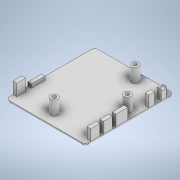
# Autodesk Inventor part: Part1
Saved by Autodesk Inventor 2022 (Build 260153000, 153)
## iProperties
Created: 2021-10-11
Part Number: Part1
Material: Generic
Document SubType Name: Modeling
Designer: Route
Density: 1 g/cm^3
Appearance: Default
Author: Route
Autodesk Inventor part; units mm, degrees
ref_plane "YZ Plane" through (0, 0, 0) normal (1, 0, 0) x (0, 1, 0)
ref_plane "XZ Plane" through (0, 0, 0) normal (0, 1, 0) x (-1, 0, 0)
ref_plane "XY Plane" through (0, 0, 0) normal (0, 0, 1) x (1, 0, 0)
sketch "Sketch1" plane through (0, 0, 0) normal (0, 1, 0) x (-1, 0, 0)
  line L0 (-30, -34) -> (30, -34)
  line L1 (30, -34) -> (30, 34)
  line L2 (30, 34) -> (-30, 34)
  line L3 (-30, 34) -> (-30, -34)
  line L4 (-30, -34) -> (30, 34) construction
  line L5 (30, -34) -> (-30, 34) construction
  line L6 (-33, 37) -> (33, 37)
  line L7 (33, 37) -> (33, -37)
  line L8 (33, -37) -> (-33, -37)
  line L9 (-33, -37) -> (-33, 37)
  line L10 (-33, 37) -> (33, -37) construction
  line L11 (33, 37) -> (-33, -37) construction
  point P0 (0, 0)
  dimension "d0" = 66
  dimension "d1" = 74
  constraints: 24 end point, 4 midpoint, 4 parallel, 2 horizontal, 2 perpendicular
  measures "d0" distance of L7.end L8.end
  measures "d1" distance of L6.end L7.end
extrude "Extrusion1" add sketch "Sketch1" along normal blind 3 contours L3 L2 L1 L0 | L6 L7 L8 L9
sketch "Sketch2" plane through (0, 3, 0) normal (0, 1, 0) x (1, 0, 0)
  line L0 (30, -34) -> (-30, -34)
  line L1 (-30, -34) -> (-30, 34)
  line L2 (-30, 34) -> (30, 34)
  line L3 (30, 34) -> (30, -34)
  line L4 (30, -34) -> (-30, 34) construction
  line L5 (-30, -34) -> (30, 34) construction
  line L6 (33, 37) -> (-33, 37) projected
  line L7 (33, -37) -> (-33, -37)
  line L8 (-33, -37) -> (-33, 37)
  line L9 (-33, 37) -> (33, 37)
  line L10 (33, 37) -> (33, -37)
  line L11 (33, -37) -> (-33, 37) construction
  line L12 (-33, -37) -> (33, 37) construction
  point P0 (0, 0)
  constraints: 24 end point, 4 midpoint, 4 parallel, 2 horizontal, 2 perpendicular
extrude "Extrusion2" add sketch "Sketch2" along normal blind 15
fillet "Fillet1" radius 3 4 edges at (33, 9, 37) (33, 9, -37) (-33, 9, -37) (-33, 9, 37)
fillet "Fillet2" radius 3 8 edges at (-32.1213, 0, 36.1213) (0, 0, 37) (32.1213, 0, 36.1213) (33, 0, 0) (32.1213, 0, -36.1213) (0, 0, -37) (-32.1213, 0, -36.1213) (-33, 0, 0)
sketch "Sketch3" plane through (0, 3, 0) normal (0, 1, 0) x (1, 0, 0)
  arc A0 (33, 34) -> (30, 37) centre (30, 34) ccw projected
  circle A1 centre (8.41, 30.19) radius 1.5
  line L0 (30, 37) -> (30, 34) projected
  circle A2 centre (26.19, 6.06) radius 1.5
  line L1 (-30, -34) -> (30, -34) projected
  circle A3 centre (-3.25, -27.65) radius 1.5
  circle A4 centre (8.41, 30.19) radius 3
  circle A5 centre (-3.25, -27.65) radius 3
  circle A6 centre (26.19, 6.06) radius 3
  point P0 (0, 0)
  dimension "d10" = 3
  dimension "d13" = 3
  dimension "d16" = 3
  dimension "d17" = 6
  dimension "d18" = 6
  dimension "d19" = 6
  constraints: 6 centre point, 3 coincident
  measures "d10" diameter of A1
  measures "d13" diameter of A2
  measures "d16" diameter of A3
  measures "d17" diameter of A4
  measures "d18" diameter of A5
  measures "d19" diameter of A6
extrude "Extrusion3" add sketch "Sketch3" along normal blind 11.4
sketch "Sketch4" plane through (0, 3, 0) normal (0, 1, 0) x (1, 0, 0)
  circle A0 centre (8.41, 30.19) radius 1.5 projected
  circle A1 centre (8.41, 30.19) radius 1.5
  circle A2 centre (26.19, 6.06) radius 1.5 projected
  circle A3 centre (26.19, 6.06) radius 1.5
  circle A4 centre (-3.25, -27.65) radius 1.5 projected
  circle A5 centre (-3.25, -27.65) radius 1.5
  point P0 (0, 0)
  constraints: 3 centre point, 3 coincident
extrude "Extrusion4" cut sketch "Sketch4" against normal blind 3
sketch "Sketch5" plane through (0, 0, 0) normal (0, -1, 0) x (1, 0, 0)
  circle A0 centre (8.41, -30.19) radius 1.5 projected
  circle A1 centre (8.41, -30.19) radius 3
  circle A2 centre (26.19, -6.06) radius 1.5 projected
  circle A3 centre (26.19, -6.06) radius 3
  circle A4 centre (-3.25, 27.65) radius 3 projected
  circle A5 centre (-3.25, 27.65) radius 3
  point P0 (0, 0)
  dimension "d24" = 6
  constraints: 3 centre point, 3 coincident
  measures "d24" diameter of A1
extrude "Extrusion5" cut sketch "Sketch5" against normal blind 2
sketch "Sketch6" plane through (-30, 3, 34) normal (1, 0, 0) x (0, 0, -1)
  line L0 (0, 0) -> (68, 0) projected
  line L1 (0, 0) -> (0, 3.6)
  line L2 (0, 15) -> (0, 0) projected
  line L3 (0, 15) -> (68, 15) projected
  line L4 (68, 0) -> (0, 0) projected
  line L5 (14.69, 3) -> (25.84, 3)
  line L6 (14.69, 3) -> (14.69, 0)
  line L7 (25.84, 3) -> (25.84, 0)
  line L8 (9.91, 0) -> (9.91, 9.529)
  line L9 (2.79, 0) -> (2.79, 9.529)
  line L10 (2.79, 9.529) -> (9.91, 9.529)
  line L11 (10.16, 0) -> (14.44, 0)
  line L12 (26.09, 0) -> (68, 0)
  line L13 (68, 0) -> (68, 15) projected
  line L14 (68, 0) -> (68, 15)
  line L15 (-3, 15) -> (0, 15) projected
  line L16 (68, 15) -> (0, 15)
  line L17 (2.54, 0) -> (2.79, 0)
  line L18 (2.54, 0) -> (2.79, 0) construction
  line L19 (10.16, 0) -> (9.91, 0)
  line L20 (10.16, 0) -> (10.41, 0) construction
  line L21 (14.44, 0) -> (14.69, 0)
  line L22 (14.44, 0) -> (14.69, 0) construction
  line L23 (26.09, 0) -> (25.84, 0)
  line L24 (26.09, 0) -> (26.34, 0) construction
  point P0 (34, -3)
  point P1 (2.79, 0)
  dimension "d27" = 3.6
  dimension "d101" = 0.25
  dimension "d102" = 0
  dimension "d103" = 0.25
  dimension "d104" = 180
  dimension "d105" = 0.25
  dimension "d106" = 0
  dimension "d107" = 0.25
  dimension "d108" = 180
  constraints: 38 end point, 8 collinear, 6 perpendicular, 4 horizontal, 2 vertical, 1 point on line
  measures "d27" distance of L0.start L1.end
  measures "d101" distance of L17.start L17.end
  measures "d102" distance between parallel lines of L17 L18
  measures "d103" distance of L19.start L19.end
  measures "d104" angle of L19 L20
  measures "d105" distance of L21.start L21.end
  measures "d106" distance between parallel lines of L21 L22
  measures "d107" distance of L23.start L23.end
  measures "d108" angle of L23 L24
sketch "Sketch7" plane through (30, 3, -34) normal (-1, 0, 0) x (0, 0, 1)
  line L0 (68, 0) -> (0, 0) projected
  line L1 (68, 0) -> (68, 3.6)
  line L2 (68, 0) -> (68, 15) projected
  line L3 (66.48, 8.861) -> (59.24, 8.861)
  line L4 (49.08, 8.861) -> (56.32, 8.861)
  line L5 (36.5, 8.861) -> (46.16, 8.861)
  line L6 (0, 15) -> (0, 0) projected
  line L7 (0, 0) -> (0, 15) projected
  line L8 (0, 3.6) -> (2.29, 3.6) construction
  line L9 (0, 15) -> (68, 15) projected
  line L10 (36.25, 15) -> (46.41, 15)
  line L11 (48.83, 15) -> (56.57, 15)
  line L12 (59, 15) -> (66.73, 15)
  line L13 (9.39, 8.1692) -> (9.39, -1.0308)
  line L14 (5.39, 8.1692) -> (5.39, 0)
  line L15 (36.5, 8.861) -> (36.5, 0)
  line L16 (46.16, 8.861) -> (46.16, 0)
  line L17 (49.08, 8.861) -> (49.08, 0)
  line L18 (56.32, 8.861) -> (56.32, 0)
  line L19 (59.24, 8.861) -> (59.24, 0)
  line L20 (66.48, 8.861) -> (66.48, 0)
  line L21 (0, 0) -> (68, 0) projected
  line L22 (9.89, 0) -> (14.761, 0)
  line L23 (14.761, 0) -> (14.761, 8.861)
  line L24 (14.761, 8.861) -> (19.341, 8.861)
  line L25 (19.341, 8.861) -> (19.341, 0)
  line L26 (5.39, 0) -> (5.64, 0)
  line L27 (5.39, 0) -> (5.64, 0) construction
  line L28 (9.89, 0) -> (9.64, 0)
  line L29 (9.89, 0) -> (10.14, 0) construction
  line L30 (14.761, 0) -> (15.011, 0)
  line L31 (14.761, 0) -> (15.011, 0) construction
  line L32 (19.841, 0) -> (19.591, 0)
  line L33 (19.841, 0) -> (20.091, 0) construction
  arc A0 (5.39, 8.1692) -> (9.39, 8.1692) centre (7.39, 8.1692) ccw
  line L34 (36.25, 0) -> (36.5, 0)
  line L35 (36.25, 0) -> (36.5, 0) construction
  line L36 (46.41, 0) -> (46.16, 0)
  line L37 (46.41, 0) -> (46.66, 0) construction
  line L38 (48.83, 0) -> (49.08, 0)
  line L39 (48.83, 0) -> (49.08, 0) construction
  line L40 (56.57, 0) -> (56.32, 0)
  line L41 (56.57, 0) -> (56.82, 0) construction
  line L42 (58.99, 0) -> (59.24, 0)
  line L43 (58.99, 0) -> (59.24, 0) construction
  line L44 (66.73, 0) -> (66.48, 0)
  line L45 (66.73, 0) -> (66.98, 0) construction
  point P0 (34, -3)
  point P1 (66.48, 0)
  point P2 (5.39, 0)
  point P3 (9.39, 0)
  point P4 (19.341, 0)
  point P5 (9.39, 0)
  point P6 (66.48, 0)
  point P7 (19.341, 0)
  dimension "d70" = 9.2
  dimension "d78" = 4.871
  dimension "d80" = 90
  dimension "d81" = 0.25
  dimension "d82" = 0
  dimension "d83" = 0.25
  dimension "d84" = 180
  dimension "d85" = 0.25
  dimension "d86" = 0
  dimension "d87" = 0.25
  dimension "d88" = 180
  dimension "d89" = 0.25
  dimension "d90" = 0
  dimension "d91" = 0.25
  dimension "d92" = 180
  dimension "d93" = 0.25
  dimension "d94" = 0
  dimension "d95" = 0.25
  dimension "d96" = 180
  dimension "d97" = 0.25
  dimension "d98" = 0
  dimension "d99" = 0.25
  dimension "d100" = 180
  constraints: 80 end point, 17 collinear, 17 horizontal, 9 perpendicular, 3 point on line, 2 point on circle, 1 centre point, 1 parallel, 1 vertical, 1 other
  measures "d70" distance of L13.start L13.end
  measures "d78" distance of L22.start L22.end
  measures "d80" angle of L23 L24
  measures "d81" distance of L26.start L26.end
  measures "d82" distance between parallel lines of L26 L27
  measures "d83" distance of L28.start L28.end
  measures "d84" angle of L28 L29
  measures "d85" distance of L30.start L30.end
  measures "d86" distance between parallel lines of L30 L31
  measures "d87" distance of L32.start L32.end
  measures "d88" angle of L32 L33
  measures "d89" distance of L34.start L34.end
  measures "d90" distance between parallel lines of L34 L35
  measures "d91" distance of L36.start L36.end
  measures "d92" angle of L36 L37
  measures "d93" distance of L38.start L38.end
  measures "d94" distance between parallel lines of L38 L39
  measures "d95" distance of L40.start L40.end
  measures "d96" angle of L40 L41
  measures "d97" distance of L42.start L42.end
  measures "d98" distance between parallel lines of L42 L43
  measures "d99" distance of L44.start L44.end
  measures "d100" angle of L44 L45
ref_plane "Work Plane1" through (30, 3, -1) normal (0, 0, -1) x (-1, 0, 0)
split body "Split1" result two bodies by plane through (30, 3, -1) normal (0, 0, -1) first body at (0.1787, 0.5, -11.4817)
move or copy body "Move Body1" bodies to move or copy 2 copy no translate (0, 0, 1.96)
combine bodies "Combine1" operation type add bodies to combine 3 2
ref_plane "Work Plane2" through (3, 3, 34) normal (1, 0, 0) x (0, 0, -1)
split body "Split2" result two bodies by plane through (3, 3, 34) normal (1, 0, 0) bodies 3 first body at (10.9943, 0.5, 1.619)
move or copy body "Move Body2" bodies to move or copy 4 copy no translate (-1.58, 0, 0)
combine bodies "Combine2" operation type add bodies to combine 4 5
extrude "Extrusion8" cut sketch "Sketch6" against normal blind 10 contours L1 L2 L3 L13 L0 L7 L5 L6 L8 L10 L9 bodies 4
extrude "Extrusion9" cut sketch "Sketch7" along normal mid plane 4 contours L0 L20 L3 L19 L18 L4 L17 L16 L5 L15 L25 L24 L23 L13 A0 L14 L6 L9 L2 L1 bodies 4
sketch "Sketch8" plane through (31.42, 3, 34) normal (0, 0, -1) x (-1, 0, 0)
  line L0 (0, 15) -> (3, 15) projected
  arc A0 (61.42, -3) -> (64.42, 0) centre (61.42, 0) ccw projected
  line L1 (0, 15) -> (64.42, 15)
  line L2 (64.42, 15) -> (64.42, 0)
  line L3 (64.42, 0) -> (0, 0)
  line L4 (0, 0) -> (0, 15)
  point P0 (31.42, -3)
  constraints: 8 end point, 2 parallel, 1 horizontal, 1 perpendicular
extrude "Extrusion10" cut sketch "Sketch8" against normal blind 10 bodies 4
sketch "Sketch9" plane through (-30, 3, -32.04) normal (0, 0, 1) x (1, 0, 0)
  line L0 (-2.2712, 0) -> (-2.2712, 15) projected
  line L1 (61.42, 0) -> (58.42, 0) projected
  line L2 (-2.2712, 15) -> (61.42, 15)
  line L3 (61.42, 15) -> (61.42, 0)
  line L4 (61.42, 0) -> (-2.2712, 0)
  line L5 (-2.2712, 0) -> (-2.2712, 15)
  point P0 (30, -3)
  constraints: 8 end point, 2 parallel, 1 horizontal, 1 perpendicular
extrude "Extrusion11" cut sketch "Sketch9" against normal blind 10 bodies 4
body "Solid4"
